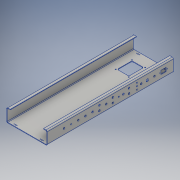
# Autodesk Inventor part: main chassis 3mm
Saved by Autodesk Inventor 2018.1 (Build 221171000, 171)
## iProperties
Created: 2018-11-28
Part Number: main chassis 3mm
Material: Aluminum 6061
Document SubType Name: Sheet Metal
Designer: RCCol
Density: 2.7 g/cm^3
Sheet Metal Rule: 3mm thick aluminum
Appearance: Aluminum - Flat
Flat Pattern Width: 37.2843 cm
Flat Pattern Length: 67.31 cm
Flat Pattern Area: 2509.61 cm^2
Sheet Metal Width: 14.679 in
Sheet Metal Length: 26.500 in
Sheet Metal Area: 388.990 in^2
Author: RCCol
Autodesk Inventor part; units mm, degrees
ref_plane "YZ Plane" through (0, 0, 0) normal (1, 0, 0) x (0, 1, 0)
ref_plane "XZ Plane" through (0, 0, 0) normal (0, 1, 0) x (-1, 0, 0)
ref_plane "XY Plane" through (0, 0, 0) normal (0, 0, 1) x (1, 0, 0)
sketch "Sketch1" plane through (0, 0, 0) normal (0, 1, 0) x (-1, 0, 0)
  line L0 (0, 0) -> (215.9, 0)
  line L1 (215.9, 0) -> (215.9, -673.1)
  line L2 (215.9, -673.1) -> (0, -673.1)
  line L3 (0, -673.1) -> (0, 0)
  dimension "d0" = 215.9
  dimension "d1" = 673.1
  measures "d0" distance of L1.end L2.end
  measures "d1" distance of L0.end L1.end
extrude "Plate1" add sketch "Sketch1" along normal blind 3
sketch "Sketch2" plane through (-212.9, 0, 0) normal (-1, 0, 0) x (0, -1, 0)
  line L0 (0, -673.1) -> (0, 0)
  line L1 (0, 0) -> (-69.85, 0)
  line L2 (-69.85, 0) -> (-69.85, -673.1)
  line L3 (-69.85, -673.1) -> (0, -673.1)
  constraints: 6 end point, 1 horizontal, 1 perpendicular, 1 vertical
edge flange "Flange1" height 69.85 angle 90 thickness 3 bend radius 3 thickness toward (-1, 0, 0) relief straight relief width 3 relief depth 1.5 edges at (-215.9, 3, -336.55) wall of the first edge with corners at (-212.9, 0, -673.1) (-212.9, 0, 0) (-212.9, 69.85, 0) (-212.9, 69.85, -673.1)
bend "Bend1"
corner "Corner1"
sketch "Sketch3" plane through (-3, 0, -673.1) normal (1, 0, 0) x (0, 1, 0)
  line L0 (0, 673.1) -> (0, 0)
  line L1 (0, 0) -> (69.85, 0)
  line L2 (69.85, 0) -> (69.85, 673.1)
  line L3 (69.85, 673.1) -> (0, 673.1)
  constraints: 6 end point, 1 horizontal, 1 perpendicular, 1 vertical
edge flange "Flange2" height 69.85 angle 90 thickness 3 bend radius 3 thickness toward (1, 0, 0) relief straight relief width 3 relief depth 1.5 edges at (0, 3, -336.55) wall of the first edge with corners at (-3, 0, 0) (-3, 0, -673.1) (-3, 69.85, -673.1) (-3, 69.85, 0)
bend "Bend2"
corner "Corner2"
sketch "Sketch4" plane through (-215.9, 66.85, 0) normal (0, 1, 0) x (-1, 0, 0)
  line L0 (0, -673.1) -> (0, 0)
  line L1 (0, 0) -> (-19.05, 0)
  line L2 (-19.05, 0) -> (-19.05, -673.1)
  line L3 (-19.05, -673.1) -> (0, -673.1)
  constraints: 6 end point, 1 horizontal, 1 perpendicular, 1 vertical
edge flange "Flange3" height 19.05 angle 90 thickness 3 bend radius 3 thickness toward (0, 1, 0) relief straight relief width 3 relief depth 1.5 corner gap 3 corner form 0 edges at (-212.9, 69.85, -336.55) (-3, 69.85, -336.55) wall of the first edge with corners at (-215.9, 66.85, -673.1) (-215.9, 66.85, 0) (-196.85, 66.85, 0) (-196.85, 66.85, -673.1)
bend "Bend3"
corner "Corner3"
sketch "Sketch11" plane through (0, 0, 0) normal (0, -1, 0) x (1, 0, 0)
  line L0 (-18.7552, -564.9839) -> (-23.6574, -564.9839)
  line L1 (-23.6574, -564.9839) -> (-23.6574, -567.0952)
  line L2 (-23.6574, -567.0952) -> (-18.7552, -567.0952)
  line L3 (-18.7552, -567.0952) -> (-18.7552, -564.9839)
  line L4 (-63.0621, -500.2637) -> (-63.0621, -503.5657)
  line L5 (-63.0621, -503.5657) -> (-59.3505, -503.5657)
  line L6 (-59.3505, -503.5657) -> (-59.3505, -500.2637)
  line L7 (-59.3505, -500.2637) -> (-63.0621, -500.2637)
  line L8 (-63.6574, -500.859) -> (-63.6574, -502.9704)
  line L9 (-63.6574, -502.9704) -> (-58.7552, -502.9704)
  line L10 (-58.7552, -502.9704) -> (-58.7552, -500.859)
  line L11 (-58.7552, -500.859) -> (-63.6574, -500.859)
  line L12 (-23.6574, -500.859) -> (-18.6753, -500.859)
  line L13 (-18.6753, -500.859) -> (-18.6753, -502.9704)
  line L14 (-18.6753, -502.9704) -> (-23.6574, -502.9704)
  line L15 (-23.6574, -502.9704) -> (-23.6574, -500.859)
  line L16 (-155.0942, -536.1747) -> (-108.3582, -536.1747)
  line L17 (-108.3582, -536.1747) -> (-108.3582, -615.6767)
  line L18 (-108.3582, -615.6767) -> (-155.0942, -615.6767)
  line L19 (-155.0942, -615.6767) -> (-155.0942, -536.1747)
  line L20 (-100.4842, -607.8027) -> (-162.9682, -607.8027)
  line L21 (-162.9682, -607.8027) -> (-162.9682, -544.0487)
  line L22 (-162.9682, -544.0487) -> (-100.4842, -544.0487)
  line L23 (-100.4842, -544.0487) -> (-100.4842, -607.8027)
  line L24 (-63.0621, -172.9161) -> (-59.3505, -172.9161)
  line L25 (-59.3505, -172.9161) -> (-59.3505, -176.2181)
  line L26 (-59.3505, -176.2181) -> (-63.0621, -176.2181)
  line L27 (-63.0621, -176.2181) -> (-63.0621, -172.9161)
  line L28 (-63.6574, -175.6228) -> (-63.6574, -173.5114)
  line L29 (-63.6574, -173.5114) -> (-58.7552, -173.5114)
  line L30 (-58.7552, -173.5114) -> (-58.7552, -175.6228)
  line L31 (-58.7552, -175.6228) -> (-63.6574, -175.6228)
  line L32 (-23.6574, -173.5114) -> (-23.6574, -175.6228)
  line L33 (-23.6574, -175.6228) -> (-18.7552, -175.6228)
  line L34 (-18.7552, -175.6228) -> (-18.7552, -173.5114)
  line L35 (-18.7552, -173.5114) -> (-23.6574, -173.5114)
  line L36 (-19.3505, -176.2181) -> (-19.3505, -172.9161)
  line L37 (-19.3505, -172.9161) -> (-23.0621, -172.9161)
  line L38 (-23.0621, -172.9161) -> (-23.0621, -176.2181)
  line L39 (-23.0621, -176.2181) -> (-19.3505, -176.2181)
  line L40 (-23.0621, -564.3885) -> (-19.3505, -564.3885)
  line L41 (-19.3505, -564.3885) -> (-19.3505, -567.6905)
  line L42 (-19.3505, -567.6905) -> (-23.0621, -567.6905)
  line L43 (-23.0621, -567.6905) -> (-23.0621, -564.3885)
  line L44 (-57.1677, -563.3964) -> (-62.0699, -563.3964)
  line L45 (-62.0699, -563.3964) -> (-62.0699, -565.5077)
  line L46 (-62.0699, -565.5077) -> (-57.1677, -565.5077)
  line L47 (-57.1677, -565.5077) -> (-57.1677, -563.3964)
  line L48 (-57.763, -566.103) -> (-57.763, -562.801)
  line L49 (-57.763, -562.801) -> (-61.4746, -562.801)
  line L50 (-61.4746, -562.801) -> (-61.4746, -566.103)
  line L51 (-61.4746, -566.103) -> (-57.763, -566.103)
  line L52 (-23.0621, -500.2637) -> (-19.3505, -500.2637)
  line L53 (-19.3505, -500.2637) -> (-19.3505, -503.5657)
  line L54 (-19.3505, -503.5657) -> (-23.0621, -503.5657)
  line L55 (-23.0621, -503.5657) -> (-23.0621, -500.2637)
  line L56 (-18.6753, -500.859) -> (-18.6753, -502.9704)
  line L57 (-18.6753, -502.9704) -> (-23.6574, -502.9704)
  line L58 (-23.6574, -502.9704) -> (-23.6574, -500.859)
  line L59 (-23.6574, -500.859) -> (-18.6753, -500.859)
  line L60 (0, -673.1) -> (0, 0.2733)
  line L61 (0, -653.7767) -> (0, -18.7767)
  line L62 (-215.9, -18.7767) -> (-215.9, -653.7767)
  line L63 (-215.9, 0.2886) -> (-215.9, -672.8114)
  circle A0 centre (-41.2063, -566.0395) radius 15.1
  arc A1 (-23.0621, -564.3885) -> (-23.6574, -564.9839) centre (-23.0621, -564.9839) ccw
  arc A2 (-18.7552, -564.9839) -> (-19.3505, -564.3885) centre (-19.3505, -564.9839) ccw
  line L64 (-19.3505, -564.3885) -> (-23.0621, -564.3885)
  arc A3 (-23.6574, -567.0952) -> (-23.0621, -567.6905) centre (-23.0621, -567.0952) ccw
  line L65 (-19.3505, -567.6905) -> (-23.0621, -567.6905)
  line L66 (-23.6574, -564.9839) -> (-23.6574, -567.0952)
  line L67 (-18.7552, -564.9839) -> (-18.7552, -567.0952)
  arc A4 (-19.3505, -567.6905) -> (-18.7552, -567.0952) centre (-19.3505, -567.0952) ccw
  arc A5 (-23.0621, -564.3885) -> (-23.6574, -564.9839) centre (-23.0621, -564.9839) ccw
  arc A6 (-18.7552, -564.9839) -> (-19.3505, -564.3885) centre (-19.3505, -564.9839) ccw
  line L68 (-19.3505, -564.3885) -> (-23.0621, -564.3885)
  arc A7 (-23.6574, -567.0952) -> (-23.0621, -567.6905) centre (-23.0621, -567.0952) ccw
  line L69 (-19.3505, -567.6905) -> (-23.0621, -567.6905)
  line L70 (-23.6574, -564.9839) -> (-23.6574, -567.0952)
  line L71 (-18.7552, -564.9839) -> (-18.7552, -567.0952)
  arc A8 (-19.3505, -567.6905) -> (-18.7552, -567.0952) centre (-19.3505, -567.0952) ccw
  circle A9 centre (-68.7342, -628.354) radius 1.651
  circle A10 centre (-26.2371, -625.179) radius 1.651
  circle A11 centre (-41.2063, -501.9147) radius 15.1
  arc A12 (-63.0621, -500.2637) -> (-63.6574, -500.859) centre (-63.0621, -500.859) ccw
  arc A13 (-58.7552, -500.859) -> (-59.3505, -500.2637) centre (-59.3505, -500.859) ccw
  line L72 (-59.3505, -500.2637) -> (-63.0621, -500.2637)
  arc A14 (-63.6574, -502.9704) -> (-63.0621, -503.5657) centre (-63.0621, -502.9704) ccw
  line L73 (-59.3505, -503.5657) -> (-63.0621, -503.5657)
  line L74 (-63.6574, -500.859) -> (-63.6574, -502.9704)
  line L75 (-58.7552, -500.859) -> (-58.7552, -502.9704)
  arc A15 (-59.3505, -503.5657) -> (-58.7552, -502.9704) centre (-59.3505, -502.9704) ccw
  arc A16 (-23.0621, -500.2637) -> (-23.6574, -500.859) centre (-23.0621, -500.859) ccw
  arc A17 (-18.7552, -500.859) -> (-19.3505, -500.2637) centre (-19.3505, -500.859) ccw
  line L76 (-19.3505, -500.2637) -> (-23.0621, -500.2637)
  arc A18 (-23.6574, -502.9704) -> (-23.0621, -503.5657) centre (-23.0621, -502.9704) ccw
  line L77 (-19.3505, -503.5657) -> (-23.0621, -503.5657)
  line L78 (-23.6574, -500.859) -> (-23.6574, -502.9704)
  line L79 (-18.7552, -500.859) -> (-18.7552, -502.9704)
  arc A19 (-19.3505, -503.5657) -> (-18.7552, -502.9704) centre (-19.3505, -502.9704) ccw
  circle A20 centre (-26.2371, -533.7645) radius 1.651
  circle A21 centre (-41.2063, -442.7924) radius 9.525
  circle A22 centre (-25.3313, -442.7924) radius 1.651
  circle A23 centre (-57.0813, -442.7924) radius 1.651
  circle A24 centre (-41.2063, -404.6924) radius 9.525
  circle A25 centre (-25.3313, -404.6924) radius 1.651
  circle A26 centre (-57.0813, -404.6924) radius 1.651
  circle A27 centre (-41.2063, -366.5924) radius 9.525
  circle A28 centre (-25.3313, -366.5924) radius 1.651
  circle A29 centre (-57.0813, -366.5924) radius 1.651
  circle A30 centre (-41.2063, -318.9674) radius 15
  circle A31 centre (-41.2063, -271.3424) radius 9.525
  circle A32 centre (-25.3313, -271.3424) radius 1.651
  circle A33 centre (-57.0813, -271.3424) radius 1.651
  circle A34 centre (-41.2063, -111.0671) radius 9.525
  circle A35 centre (-25.3313, -111.0671) radius 1.651
  circle A36 centre (-57.0813, -111.0671) radius 1.651
  circle A37 centre (-41.2063, -66.6171) radius 9.525
  circle A38 centre (-25.3313, -66.6171) radius 1.651
  circle A39 centre (-57.0813, -66.6171) radius 1.651
  line L80 (-215.9, -672.8114) -> (0, -673.1)
  line L81 (-215.9, 0.2886) -> (0, 0.2733)
  line L82 (-162.9682, -607.8027) -> (-162.9682, -544.0487)
  arc A40 (-155.0942, -536.1747) -> (-162.9682, -544.0487) centre (-155.0942, -544.0487) ccw
  line L83 (-155.0942, -536.1747) -> (-108.3582, -536.1747)
  arc A41 (-100.4842, -544.0487) -> (-108.3582, -536.1747) centre (-108.3582, -544.0487) ccw
  line L84 (-100.4842, -544.0487) -> (-100.4842, -607.8027)
  arc A42 (-108.3582, -615.6767) -> (-100.4842, -607.8027) centre (-108.3582, -607.8027) ccw
  line L85 (-108.3582, -615.6767) -> (-155.0942, -615.6767)
  arc A43 (-162.9682, -607.8027) -> (-155.0942, -615.6767) centre (-155.0942, -607.8027) ccw
  circle A44 centre (-96.8012, -619.6137) radius 2.7813
  circle A45 centre (-96.8012, -532.2377) radius 2.7813
  circle A46 centre (-166.6512, -619.6137) radius 2.7813
  circle A47 centre (-166.6512, -532.2377) radius 2.7813
  circle A48 centre (-41.2063, -174.5671) radius 15.1
  arc A49 (-63.0621, -172.9161) -> (-63.6574, -173.5114) centre (-63.0621, -173.5114) ccw
  arc A50 (-58.7552, -173.5114) -> (-59.3505, -172.9161) centre (-59.3505, -173.5114) ccw
  line L86 (-59.3505, -172.9161) -> (-63.0621, -172.9161)
  arc A51 (-63.6574, -175.6228) -> (-63.0621, -176.2181) centre (-63.0621, -175.6228) ccw
  line L87 (-59.3505, -176.2181) -> (-63.0621, -176.2181)
  line L88 (-63.6574, -173.5114) -> (-63.6574, -175.6228)
  line L89 (-58.7552, -173.5114) -> (-58.7552, -175.6228)
  arc A52 (-59.3505, -176.2181) -> (-58.7552, -175.6228) centre (-59.3505, -175.6228) ccw
  arc A53 (-23.0621, -172.9161) -> (-23.6574, -173.5114) centre (-23.0621, -173.5114) ccw
  arc A54 (-18.7552, -173.5114) -> (-19.3505, -172.9161) centre (-19.3505, -173.5114) ccw
  line L90 (-19.3505, -172.9161) -> (-23.0621, -172.9161)
  arc A55 (-23.6574, -175.6228) -> (-23.0621, -176.2181) centre (-23.0621, -175.6228) ccw
  line L91 (-19.3505, -176.2181) -> (-23.0621, -176.2181)
  line L92 (-23.6574, -173.5114) -> (-23.6574, -175.6228)
  line L93 (-18.7552, -173.5114) -> (-18.7552, -175.6228)
  arc A56 (-19.3505, -176.2181) -> (-18.7552, -175.6228) centre (-19.3505, -175.6228) ccw
  circle A57 centre (-30.7594, -9.2517) radius 1.5875
  circle A58 centre (-185.1406, -9.2517) radius 1.5875
  circle A59 centre (-177.8, -9.2517) radius 2.667
  circle A60 centre (-170.4594, -9.2517) radius 1.5875
  circle A61 centre (-45.4406, -9.2517) radius 1.5875
  circle A62 centre (-38.1, -9.2517) radius 2.667
  circle A63 centre (-185.1406, -663.4383) radius 1.5875
  circle A64 centre (-177.8, -663.4383) radius 2.667
  circle A65 centre (-170.4594, -663.4383) radius 1.5875
  circle A66 centre (-45.4406, -663.4383) radius 1.5875
  circle A67 centre (-38.1, -663.4383) radius 2.667
  circle A68 centre (-30.7594, -663.4383) radius 1.5875
  circle A69 centre (-155.0942, -607.8027) radius 7.874
  circle A70 centre (-155.0942, -544.0487) radius 7.874
  circle A71 centre (-108.3582, -544.0487) radius 7.874
  circle A72 centre (-108.3582, -607.8027) radius 7.874
  circle A73 centre (-23.0621, -564.9839) radius 0.5953
  circle A74 centre (-23.0621, -567.0952) radius 0.5953
  circle A75 centre (-19.3505, -567.0952) radius 0.5953
  circle A76 centre (-19.3505, -564.9839) radius 0.5953
  circle A77 centre (-57.763, -563.3964) radius 0.5953
  line L94 (-57.1677, -563.3964) -> (-57.1677, -565.5077)
  arc A78 (-57.763, -566.103) -> (-57.1677, -565.5077) centre (-57.763, -565.5077) ccw
  line L95 (-57.763, -562.801) -> (-61.4746, -562.801)
  arc A79 (-61.4746, -562.801) -> (-62.0699, -563.3964) centre (-61.4746, -563.3964) ccw
  circle A80 centre (-61.4746, -563.3964) radius 0.5953
  line L96 (-57.763, -566.103) -> (-61.4746, -566.103)
  line L97 (-62.0699, -563.3964) -> (-62.0699, -565.5077)
  arc A81 (-57.1677, -563.3964) -> (-57.763, -562.801) centre (-57.763, -563.3964) ccw
  arc A82 (-62.0699, -565.5077) -> (-61.4746, -566.103) centre (-61.4746, -565.5077) ccw
  circle A83 centre (-57.763, -565.5077) radius 0.5953
  circle A84 centre (-61.4746, -565.5077) radius 0.5953
  circle A85 centre (-63.0621, -500.859) radius 0.5953
  circle A86 centre (-59.3505, -500.859) radius 0.5953
  circle A87 centre (-59.3505, -502.9704) radius 0.5953
  circle A88 centre (-63.0621, -502.9704) radius 0.5953
  circle A89 centre (-23.0621, -500.859) radius 0.5953
  circle A90 centre (-23.0621, -502.9704) radius 0.5953
  circle A91 centre (-19.3505, -502.9704) radius 0.5953
  circle A92 centre (-19.3505, -500.859) radius 0.5953
  circle A93 centre (-63.0621, -173.5114) radius 0.5953
  circle A94 centre (-59.3505, -173.5114) radius 0.5953
  circle A95 centre (-59.3505, -175.6228) radius 0.5953
  circle A96 centre (-63.0621, -175.6228) radius 0.5953
  circle A97 centre (-23.0621, -173.5114) radius 0.5953
  circle A98 centre (-23.0621, -175.6228) radius 0.5953
  circle A99 centre (-19.3505, -175.6228) radius 0.5953
  circle A100 centre (-19.3505, -173.5114) radius 0.5953
  point P0 (0, 0)
  constraints: 196 end point, 101 centre point, 64 point on circle
extrude "Cut4" cut sketch "Sketch11" against normal blind 3 contours A76 L41 L0 | L0 L41 A2 | L3 A75 L41 A76 | L41 A76 L0 | L0 A76 L41 | A4 L41 L2 | L2 L41 A75 | A76 L0 A73 L40 | L41 A75 L2 A74 L43 A73 L0 A76 | L41 A75 L2 | L2 A75 L41 | L42 A74 L2 A75 | A73 L0 L43 | L43 L0 A1 | A73 L43 L0 | A3 L2 L43 | L43 L2 A74 | L43 A73 L0 | A73 L43 A74 L1 | L2 L43 A74 | L2 A74 L43 | A85 L11 L4 | L4 L11 A12 | L7 A86 L11 A85 | L11 A85 L4 | L4 A85 L11 | A13 L11 L6 | L6 L11 A86 | A85 L4 A88 L8 | L11 A86 L6 A87 L9 A88 L4 A85 | L11 A86 L6 | L6 A86 L11 | L10 A87 L6 A86 | A88 L4 L9 | L9 L4 A14 | A88 L9 L4 | A15 L6 L9 | L9 L6 A87 | L9 A88 L4 | A88 L9 A87 L5 | L6 L9 A87 | L6 A87 L9 | A92 L53 L12 | L12 L53 A17 | L12 L13 L14 L79 | L79 A91 L53 A92 | L53 A92 L12 | L12 A92 L53 | A92 L12 A89 L52 | A19 L53 L14 | L14 L53 A91 | L53 A91 L14 A90 L55 A89 L12 A92 | A89 L12 L55 | L55 L12 A16 | L53 A91 L14 | L14 A91 L53 | L54 A90 L14 A91 | A89 L55 L12 | L55 A89 L12 | A89 L55 A90 L15 | A18 L14 L55 | L55 L14 A90 | A90 L55 L14 | L14 L55 A90 | A70 L22 L19 | L19 L22 A40 | L16 A71 L22 A70 | A41 L22 L17 | L17 L22 A71 | L22 A70 L19 | L19 A70 L22 | A70 L19 A69 L21 | L22 A71 L17 A72 L20 A69 L19 A70 | L22 A71 L17 | L17 A71 L22 | L23 A72 L17 A71 | A69 L19 L20 | L20 L19 A43 | A42 L17 L20 | L20 L17 A72 | A69 L20 L19 | L20 A69 L19 | A69 L20 A72 L18 | L17 L20 A72 | L17 A72 L20 | A93 L29 L27 | L27 L29 A49 | L24 A94 L29 A93 | A50 L29 L25 | L25 L29 A94 | L29 A93 L27 | L27 A93 L29 | A93 L27 A96 L28 | L29 A94 L25 A95 L31 A96 L27 A93 | L29 A94 L25 | L25 A94 L29 | L30 A95 L25 A94 | A96 L27 L31 | L31 L27 A51 | A52 L25 L31 | L31 L25 A95 | A96 L31 L27 | L31 A96 L27 | A96 L31 A95 L26 | L25 L31 A95 | L25 A95 L31 | A97 L38 A98 L32 | A53 L38 L35 | L35 L38 A97 | A98 L38 L33 | L33 L38 A55 | L38 A97 L35 | L35 A97 L38 | L37 A100 L35 A97 | A97 L35 A100 L36 A99 L33 A98 L38 | L38 A98 L33 | L33 A98 L38 | A98 L33 A99 L39 | A54 L35 L36 | L36 L35 A100 | A99 L33 L36 | L36 L33 A56 | L35 L36 A100 | L35 A100 L36 | L34 A99 L36 A100 | A99 L36 L33 | L36 A99 L33 | A77 L48 L44 | L44 L48 A77 | L47 A83 L48 A77 | L48 A77 L44 | L44 A77 L48 | A78 L48 L46 | L46 L48 A83 | A77 L44 A80 L49 | L48 A83 L46 A84 L50 A80 L44 A77 | L48 A83 L46 | L46 A83 L48 | L51 A84 L46 A83 | A80 L44 L50 | L50 L44 A79 | A80 L50 L44 | A82 L46 L50 | L50 L46 A84 | L50 A80 L44 | A80 L50 A84 L45 | L46 L50 A84 | L46 A84 L50 | A0 | A9 | A10 | A11 | A20 | A21 | A22 | A23 | A24 | A25 | A26 | A27 | A28 | A29 | A30 | A31 | A32 | A33 | A34 | A35 | A36 | A37 | A38 | A39 | A44 | A45 | A46 | A47 | A48 | A57 | A58 | A59 | A60 | A61 | A62 | A63 | A64 | A65 | A66 | A67 | A68
sketch "Sketch12" plane through (0, 6, 0) normal (1, 0, 0) x (0, 0, -1)
  line L0 (0, -6) -> (0, 63.85)
  line L1 (0, 63.85) -> (673.1, 63.85)
  line L2 (673.1, 63.85) -> (673.1, -6)
  line L3 (673.1, -6) -> (0, -6)
  line L4 (634.5201, 38.8469) -> (634.5201, 19.0031)
  line L5 (634.5201, 19.0031) -> (606.8239, 19.0031)
  line L6 (606.8239, 19.0031) -> (606.8239, 38.8469)
  line L7 (606.8239, 38.8469) -> (634.5201, 38.8469)
  line L8 (528.4218, 32.2343) -> (539.8518, 32.2343)
  arc A0 (539.8518, 32.2343) -> (528.4218, 32.2343) centre (534.1368, 28.925) ccw
  arc A1 (539.8518, 32.2343) -> (528.4218, 32.2343) centre (534.1368, 28.925) ccw
  line L9 (528.4218, 32.2343) -> (528.4218, 25.6157)
  arc A2 (528.4218, 25.6157) -> (539.8518, 25.6157) centre (534.1368, 28.925) ccw
  line L10 (539.8518, 25.6157) -> (539.8518, 32.2343)
  line L11 (528.4218, 32.2343) -> (528.4218, 25.6157)
  line L12 (528.4218, 25.6157) -> (539.8518, 25.6157)
  line L13 (539.8518, 25.6157) -> (539.8518, 32.2343)
  arc A3 (539.8518, 32.2343) -> (528.4218, 32.2343) centre (534.1368, 28.925) ccw
  line L14 (528.4218, 32.2343) -> (528.4218, 25.6157)
  line L15 (528.4218, 25.6157) -> (539.8518, 25.6157)
  line L16 (539.8518, 25.6157) -> (539.8518, 32.2343)
  arc A4 (539.8518, 32.2343) -> (528.4218, 32.2343) centre (534.1368, 28.925) ccw
  line L17 (539.8518, 25.6157) -> (539.8518, 32.2343)
  line L18 (539.8518, 32.2343) -> (528.4218, 32.2343)
  line L19 (528.4218, 32.2343) -> (528.4218, 25.6157)
  line L20 (528.4218, 25.6157) -> (539.8518, 25.6157)
  line L21 (539.8518, 25.6157) -> (539.8518, 32.2343)
  circle A5 centre (242.1644, 28.925) radius 4.7625
  circle A6 centre (242.1644, 28.925) radius 4.7625
  circle A7 centre (89.7644, 28.925) radius 4.7625
  circle A8 centre (165.9644, 28.925) radius 4.7625
  circle A9 centre (278.5826, 41.625) radius 4.7625
  circle A10 centre (278.5826, 16.225) radius 4.7625
  circle A11 centre (278.5826, 16.225) radius 4.7625
  circle A12 centre (278.5826, 41.625) radius 4.7625
  circle A13 centre (406.55, 28.925) radius 4.7625
  circle A14 centre (406.55, 28.925) radius 4.7625
  circle A15 centre (572.3167, 28.925) radius 4.7625
  circle A16 centre (572.3167, 28.925) radius 4.7625
  circle A17 centre (204.0644, 28.925) radius 4.7625
  circle A18 centre (204.0644, 28.925) radius 4.7625
  circle A19 centre (382.0232, 28.8879) radius 3.2004
  circle A20 centre (591.3667, 28.925) radius 1.016
  circle A21 centre (553.2667, 28.925) radius 1.016
  circle A22 centre (585.7871, 42.3954) radius 1.016
  circle A23 centre (572.3167, 47.975) radius 1.016
  circle A24 centre (558.8464, 42.3954) radius 1.016
  circle A25 centre (479.5509, 13.05) radius 3.2385
  circle A26 centre (479.5509, 28.925) radius 3.2385
  circle A27 centre (479.5509, 44.8) radius 3.2385
  circle A28 centre (501.7518, 28.925) radius 4.7625
  circle A29 centre (501.7518, 28.925) radius 4.7625
  circle A30 centre (315.1281, 28.925) radius 4.7625
  circle A31 centre (315.1281, 28.925) radius 4.7625
  circle A32 centre (350.2038, 41.625) radius 4.7625
  circle A33 centre (350.2038, 16.225) radius 4.7625
  circle A34 centre (350.2038, 16.225) radius 4.7625
  circle A35 centre (350.2038, 41.625) radius 4.7625
  circle A36 centre (127.8644, 28.925) radius 3.2004
  circle A37 centre (436.7125, 41.625) radius 4.7625
  circle A38 centre (436.7125, 16.225) radius 4.7625
  circle A39 centre (436.7125, 16.225) radius 4.7625
  circle A40 centre (436.7125, 41.625) radius 4.7625
  circle A41 centre (600.8282, 28.925) radius 1.651
  circle A42 centre (640.5157, 28.925) radius 1.651
  arc A43 (528.4218, 25.6157) -> (539.8518, 25.6157) centre (534.1368, 28.925) ccw
  line L22 (539.8518, 25.6157) -> (528.4218, 25.6157)
  line L23 (528.4218, 25.6157) -> (528.4218, 32.2343)
  line L24 (528.4218, 32.2343) -> (539.8518, 32.2343)
  line L25 (539.8518, 32.2343) -> (539.8518, 25.6157)
  arc A44 (528.4218, 25.6157) -> (539.8518, 25.6157) centre (534.1368, 28.925) ccw
  point P0 (0, -6)
  constraints: 52 end point, 45 centre point, 15 point on circle, 2 parallel, 1 coincident, 1 concentric, 1 horizontal, 1 perpendicular, 1 point on line
extrude "Cut5" cut sketch "Sketch12" against normal blind 3 contours L4 L5 L6 L7 | A0 L8 | L8 L10 L12 L9 | L12 A2 | A5 | A7 | A8 | A9 | A10 | A13 | A15 | A17 | A19 | A25 | A26 | A27 | A28 | A30 | A32 | A33 | A36 | A37 | A38 | A41 | A42
equation "\"d53\" = Thickness"
equation "\"d55\" = Thickness"
equation "\"d2\" = Thickness"
equation "\"d3\" = BendReliefWidth"
equation "\"d4\" = BendReliefDepth"
equation "\"d5\" = MinimumRemnant"
equation "\"d6\" = TransitionRadius"
equation "\"d9\" = BendRadius"
equation "\"d10\" = CornerReliefSize"
equation "\"d11\" = GapSize"
equation "\"d12\" = JacobiRadiusSize"
equation "\"d13\" = BendReliefWidth"
equation "\"d14\" = BendReliefDepth"
equation "\"d15\" = MinimumRemnant"
equation "\"d16\" = TransitionRadius"
equation "\"d19\" = BendRadius"
equation "\"d20\" = CornerReliefSize"
equation "\"d21\" = GapSize"
equation "\"d22\" = JacobiRadiusSize"
equation "\"d23\" = BendReliefWidth"
equation "\"d24\" = BendReliefDepth"
equation "\"d25\" = MinimumRemnant"
equation "\"d26\" = TransitionRadius"
equation "\"d29\" = BendRadius"
equation "\"d30\" = CornerReliefSize"
equation "\"d31\" = GapSize"
equation "\"d32\" = JacobiRadiusSize"
equation "\"BendRadius\" = Thickness"
equation "\"BendReliefWidth\" = Thickness"
equation "\"BendReliefDepth\" = 0.5 * Thickness"
equation "\"CornerReliefSize\" = 4 * Thickness"
equation "\"MinimumRemnant\" = 2 * Thickness"
equation "\"TransitionRadius\" = BendRadius"
equation "\"JacobiRadiusSize\" = BendRadius"
equation "\"Thickness\" = 3"
equation "\"GapSize\" = 3"
body "Solid1"
